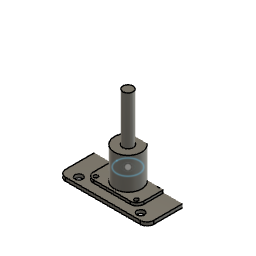
assembly (Autodesk Fusion 360 design; units mm, degrees)
Autodesk Fusion 360 part; units mm, degrees
sketch "Sketch1" plane through (0, 0, 0) normal (0, 1, 0) x (1, 0, 0) in component "base v3"
  line L0 (0, 0) -> (130.3022, 0)
  line L1 (130.3022, 0) -> (130.3022, -74.3286)
  line L2 (130.3022, -74.3286) -> (0, -74.3286)
  line L3 (0, -74.3286) -> (0, 0)
  circle A0 centre (19.4502, -10.1604) radius 5.6189
  circle A1 centre (110.8519, -10.1604) radius 5.6189
  circle A2 centre (19.4502, -64.1683) radius 5.6189
  circle A3 centre (110.8519, -64.1683) radius 5.6189
  circle A4 centre (35.2621, -19.7238) radius 2.9659
  circle A5 centre (95.0401, -19.7238) radius 2.9659
  circle A6 centre (35.2621, -54.6049) radius 2.9659
  circle A7 centre (95.0401, -54.6049) radius 2.9659
  line L4 (35.2621, -54.6049) -> (37.8238, -53.1101) construction
  line L5 (92.4783, -21.2186) -> (95.0401, -19.7238) construction
  line L6 (95.0401, -54.6049) -> (92.4783, -53.1101) construction
  line L7 (37.8238, -21.2186) -> (35.2621, -19.7238) construction
  constraint horizontal L0
  constraint vertical L1
  constraint horizontal L2
  constraint vertical L3
  constraint coincident L0.start L3.end
  constraint coincident A4.centre L7.end
  constraint coincident A5 L5.start
  constraint collinear L4 L5
  constraint coincident A4 L7.start
  constraint collinear L6 L7
  constraint coincident A6 L4.end
  constraint coincident A7 L6.end
extrude "Extrude1" add sketch "Sketch1" along normal blind 5 contours L0 L1 L2 L3 | A4 | A5 | A6 | A7 makes body 1 in component "base v3"
fillet "Fillet1" radius 10 4 edges at (0, 2.5, 74.3286) (0, 2.5, 0) (130.3022, 2.5, 74.3286) (130.3022, 2.5, 0) on bodies 1 in component "base v3"
extrude "Extrude2" cut sketch "Sketch1" along normal blind 5 contours A4 | A5 | A6 | A7 bodies 1 in component "base v3"
sketch "Sketch1 (2)" plane through (0, 0, 0) normal (0, 1, 0) x (1, 0, 0) in component "Cam gear base v4"
  line L0 (0, 0) -> (59.778, 0)
  line L1 (59.778, 0) -> (59.778, -34.881)
  line L2 (59.778, -34.881) -> (0, -34.881)
  line L3 (0, -34.881) -> (0, 0)
  circle A0 centre (0, 0) radius 3
  line L4 (29.889, 0) -> (29.889, -34.881) construction
  line L5 (0, -17.4405) -> (59.778, -17.4405) construction
  circle A1 centre (0, -34.881) radius 3
  circle A2 centre (59.778, 0) radius 3
  circle A3 centre (59.778, -34.881) radius 3
  line L6 (67.0978, -41.2769) -> (-7.3198, -41.2769)
  line L7 (-7.3198, -41.2769) -> (-7.3198, 6.3959)
  line L8 (-7.3198, 6.3959) -> (67.0978, 6.3959)
  line L9 (67.0978, 6.3959) -> (67.0978, -41.2769)
  line L10 (67.0978, -41.2769) -> (-7.3198, 6.3959) construction
  line L11 (-7.3198, -41.2769) -> (67.0978, 6.3959) construction
  point P0 (29.889, -17.4405)
  dimension "d1_3" = 59.778
  dimension "d2_3" = 34.881
  dimension "d3_3" = 6
  constraint horizontal L0
  constraint vertical L1
  constraint horizontal L2
  constraint vertical L3
  constraint coincident L0.start L3.end
  constraint midpoint L0 L4.start
  constraint midpoint L2 L4.end
  constraint midpoint L3 L5.start
  constraint midpoint L1 L5.end
  constraint symmetric A0 L5 A1
  constraint symmetric A0 L4 A2
  constraint symmetric L4 A1 A3
  constraint horizontal L6
  constraint perpendicular L6 L7
  constraint parallel L6 L8
  constraint parallel L7 L9
  constraint coincident L10 P0
  constraint coincident L11 P0
  constraint midpoint L4 P0
  measures "d1_3" distance of L0.start L0.end
  measures "d2_3" distance of L0.end L1.end
  measures "d3_3" diameter of A0
extrude "Extrude1'" add sketch "Sketch1 (2)" along normal blind 4 separate body contours L0 L1 L2 L3 A0 A1 A2 A3 | L6 L7 L8 L9 makes body 2 in component "Cam gear base v4"
fillet "Fillet1'" radius 10 4 edges at (67.0978, 2, 41.2769) (67.0978, 2, -6.3959) (-7.3198, 2, 41.2769) (-7.3198, 2, -6.3959) on bodies 2 in component "Cam gear base v4"
sketch "Sketch2" plane through (0, 4, 0) normal (0, 1, 0) x (-1, 0, 0) in component "Cam gear base v4"
  arc A0 (-2.6802, -6.3959) -> (7.3198, 3.6041) centre (-2.6802, 3.6041) ccw
  line L0 (7.3198, 3.6041) -> (7.3198, 31.2769)
  arc A1 (7.3198, 31.2769) -> (-2.6802, 41.2769) centre (-2.6802, 31.2769) ccw
  line L1 (-2.6802, 41.2769) -> (-57.0978, 41.2769)
  arc A2 (-57.0978, 41.2769) -> (-67.0978, 31.2769) centre (-57.0978, 31.2769) ccw
  line L2 (-67.0978, 31.2769) -> (-67.0978, 3.6041)
  arc A3 (-67.0978, 3.6041) -> (-57.0978, -6.3959) centre (-57.0978, 3.6041) ccw
  line L3 (-57.0978, -6.3959) -> (-2.6802, -6.3959)
  circle A4 centre (0, 0) radius 3
  circle A5 centre (-59.778, 0) radius 3
  circle A6 centre (0, 34.881) radius 3
  circle A7 centre (-59.778, 34.881) radius 3
  line L4 (-29.889, -6.3959) -> (-29.889, 41.2769) construction
  line L5 (7.3198, 17.4405) -> (-67.0978, 17.4405) construction
  circle A8 centre (-29.889, 17.4405) radius 20
  circle A9 centre (-29.889, 17.4405) radius 17.5
  line L6 (-17.85, 18.4405) -> (-41.928, 18.4405)
  arc A10 (-41.928, 18.4405) -> (-41.928, 16.4405) centre (-41.928, 17.4405) ccw
  line L7 (-41.928, 16.4405) -> (-17.85, 16.4405)
  arc A11 (-17.85, 16.4405) -> (-17.85, 18.4405) centre (-17.85, 17.4405) ccw
  line L8 (-17.85, 17.4405) -> (-41.928, 17.4405) construction
  line L9 (-17.85, 16.4405) -> (-17.85, 18.4405)
  line L10 (-41.928, 16.4405) -> (-41.928, 18.4405)
  point P0 (-29.889, 17.4405)
  dimension "d8_1" = 40
  dimension "d9" = 35
  dimension "d10" = 2
  constraint midpoint L3 L4.start
  constraint midpoint L1 L4.end
  constraint midpoint L0 L5.start
  constraint midpoint L2 L5.end
  constraint midpoint L5 P0
  constraint concentric A8 A9
  constraint tangent L6 A10
  constraint tangent A10 L7
  constraint parallel L6 L7
  constraint tangent L7 A11
  constraint tangent L6 A11
  constraint coincident L5 A10.centre
  constraint perpendicular L4 L8
  constraint coincident P0 A8.centre
  constraint midpoint L8 P0
  measures "d8_1" diameter of A8
  measures "d9" diameter of A9
  measures "d10" diameter of A10
extrude "Extrude2'" add sketch "Sketch2" along normal blind 2 contours L6 L7 L9 L10 bodies 2 in component "Cam gear base v4"
sketch "Sketch3" plane through (0, 0, 18.4405) normal (0, 0, 1) x (1, 0, 0) in component "Cam gear base v4"
  line L0 (17.85, 4) -> (41.928, 4)
  line L1 (41.928, 4) -> (41.928, 6)
  line L2 (41.928, 6) -> (17.85, 6)
  line L3 (17.85, 6) -> (17.85, 4)
  arc A0 (41.928, 6) -> (17.85, 6) centre (29.889, 6) ccw
  constraint midpoint L2 A0.centre
extrude "Extrude3" add sketch "Sketch3" against normal blind 2 contours L2 A0 bodies 2 in component "Cam gear base v4"
sketch "Sketch4" plane through (0, 0, 18.4405) normal (0, 0, 1) x (1, 0, 0) in component "Cam gear base v4"
  line L0 (17.85, 4) -> (41.928, 4)
  line L1 (41.928, 4) -> (41.928, 6)
  arc A0 (41.928, 6) -> (17.85, 6) centre (29.889, 6) ccw
  line L2 (17.85, 6) -> (17.85, 4)
  circle A1 centre (29.889, 15.2616) radius 1.4686
extrude "Extrude4" cut sketch "Sketch4" against normal blind 2 contours A1 bodies 2 in component "Cam gear base v4"
extrude "Extrude5" add sketch "Sketch2" along normal blind 45 contours A8 bodies 2 in component "Cam gear base v4"
sketch "Sketch5" plane through (0, 49, 0) normal (0, 1, 0) x (-1, 0, 0) in component "Cam gear base v4"
  circle A0 centre (-29.889, 17.4405) radius 17.5
  circle A1 centre (-29.889, 17.4405) radius 20
  circle A2 centre (-29.889, 17.4405) radius 20
  constraint concentric A0 A2
extrude "Extrude6" add sketch "Sketch5" along normal blind 2 contours A0 | A1 A2 bodies 2 in component "Cam gear base v4"
sketch "Sketch6" plane through (0, 51, 0) normal (0, 1, 0) x (-1, 0, 0) in component "Cam gear base v4"
  circle A0 centre (-29.889, 17.4405) radius 20
  circle A1 centre (-29.889, 17.4405) radius 8
  dimension "d21" = 16
  constraint concentric A0 A1
  measures "d21" diameter of A1
extrude "Extrude7" cut sketch "Sketch6" against normal blind 2 contours A1 bodies 2 in component "Cam gear base v4"
sketch "Sketch1 (3)" plane through (0, 0, 0) normal (0, 1, 0) x (1, 0, 0)
  ellipse E0 centre (0, 0) end of major axis (10, 0) minor radius 3.5
  line L0 (-10, 0) -> (10, 0)
  line L1 (0, -3.5) -> (0, 3.5)
  circle A0 centre (0, 0) radius 1
  dimension "d1_2" = 7
  dimension "d2_2" = 2
  dimension "d3_2" = 10
  constraint coincident E0.centre A0.centre
  constraint horizontal L0
  constraint coincident E0 L0.start
  constraint coincident E0 L0.end
  constraint coincident E0 L1.start
  constraint coincident E0 L1.end
  measures "d2_2" diameter of A0
  measures "d3_2" distance of E0
extrude "Extrude1''" add sketch "Sketch1 (3)" along normal blind 3 separate body contours E0 L0 L1 A0 | E0 L0 L1 A0 | E0 L0 L1 A0 | E0 L0 L1 A0 makes body 3
sketch "Sketch1 (4)" plane through (0, 0, 0) normal (0, 1, 0) x (1, 0, 0) in component "Brush guide v4"
  circle A0 centre (0, 0) radius 17.5
  dimension "d1_4" = 35
  constraint coincident A0.centre origin
  measures "d1_4" diameter of A0
extrude "Extrude1'''" add sketch "Sketch1 (4)" along normal blind 3 separate body makes body 4 in component "Brush guide v4"
fillet "Fillet1''" radius 1 1 edges at (-16.3157, 3, 6.3283) on bodies 4 in component "Brush guide v4"
fillet "Fillet2" radius 1 1 edges at (-16.3157, 0, 6.3283) on bodies 4 in component "Brush guide v4"
sketch "Sketch2 (2)" plane through (0, 3, 0) normal (0, 1, 0) x (-1, 0, 0) in component "Brush guide v4"
  circle A0 centre (0, 0) radius 16.5
  circle A1 centre (0, 0) radius 7.5
  dimension "d8_2" = 15
  constraint coincident A0.centre A1.centre
  measures "d8_2" diameter of A1
extrude "Extrude2''" add sketch "Sketch2 (2)" along normal blind 100 contours A1 bodies 4 in component "Brush guide v4"
ref_plane "WorkPlane1" through (0, 23, 0) normal (0, 1, 0) x (-1, 0, 0) in component "Brush guide v4"
sketch "Sketch6 (2)" plane through (0, 3, 0) normal (0, 1, 0) x (-1, 0, 0) in component "Brush guide v4"
  circle A0 centre (0, 0) radius 7.5
  circle A1 centre (0, 0) radius 16.5
  circle A2 centre (0, 0) radius 16.5
  constraint concentric A0 A2
ref_plane "WorkPlane2" through (0, 6, 0) normal (0, 1, 0) x (-1, 0, 0) in component "Brush guide v4"
coil "CoilPrimitive3" add diameter 25 section circle size 2 on centre turns 8 pitch 2.5 right hand placed x (1, 0, 0) y (0, 0, -1) z (0, 1, 0) at (0, 6, 0) separate body makes body 5 in component "Brush guide v4"
